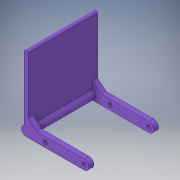
# Autodesk Inventor part: Mouth-Height-Lever-front
Saved by Autodesk Inventor 2018.3 (Build 223284000, 284)
## iProperties
Created: 2018-05-17
Part Number: Mouth-Height-Lever-front
Material: Generisch
Document SubType Name: Modeling
Designer: JochenAlt
Density: 1 g/cm^3
Appearance: Violett
Author: JochenAlt
Autodesk Inventor part; units mm, degrees
ref_plane "YZ Plane" through (0, 0, 0) normal (1, 0, 0) x (0, 1, 0)
ref_plane "XZ Plane" through (0, 0, 0) normal (0, 1, 0) x (-1, 0, 0)
ref_plane "XY Plane" through (0, 0, 0) normal (0, 0, 1) x (1, 0, 0)
sketch "Skizze4" plane through (0, 0, 0) normal (0, 1, 0) x (-1, 0, 0)
  line L0 (-32.5, 2.5) -> (-2.5, 2.5) construction
  line L1 (0, -10.2627) -> (0, 44.0763) construction
  line L2 (-42, 0) -> (7, 0) construction
  circle A0 centre (-32.5, 0) radius 2.5
  circle A1 centre (-32.5, 0) radius 1
  circle A2 centre (-2.5, 0) radius 2.5
  line L3 (-2.5, -2.5) -> (-32.5, -2.5) construction
  circle A3 centre (-12.5, 0) radius 2.5
  line L4 (-32.5, 2.5) -> (-12.5, 2.5)
  line L5 (-12.5, 2.5) -> (-7.7873, 2.5)
  line L6 (-32.5, -2.5) -> (-12.5, -2.5)
  line L7 (-12.5, -2.5) -> (-7.7873, -2.5)
  line L8 (-1.5, 2.2913) -> (-1.5, 35.3136)
  arc A4 (-1.5, 35.3136) -> (-3.5, 35.3136) centre (-2.5, 35.3136) ccw
  circle A5 centre (-12.5, 0) radius 1
  line L9 (-7.7873, 2.5) -> (-3.5, 6.3118)
  line L10 (-3.5, 6.3118) -> (-3.5, 35.3136)
  line L11 (-7.7873, 2.5) -> (-2.5, 2.5)
  line L12 (-7.7873, 2.5) -> (-7.7873, -2.5)
  line L13 (-7.7873, -2.5) -> (-2.5, -2.5)
  line L14 (-3.5, 6.3118) -> (-3.5, 2.2913)
  point P0 (0, 0)
  dimension "d28" = 2
  dimension "d30" = 10
  dimension "d32" = 20
  dimension "d33" = 5
  dimension "d35" = 5
  constraints: 26 end point, 16 point on circle, 9 tangent, 6 centre point, 5 parallel, 3 horizontal, 2 coincident, 2 vertical, 1 collinear, 1 equal radius, 2 other
  measures "d28" diameter of A1
  measures "d30" distance of A2.centre A3.centre
  measures "d32" distance of A3.centre A0.centre
  measures "d33" distance between parallel lines of L6 L4
  measures "d35" diameter of A2
extrude "Extrusion6" add sketch "Skizze4" along normal mid plane 36
extrude "Extrusion7" cut sketch "Skizze4" along normal mid plane 31 contours A0 | A0 L4 A3 L6 | L5 L12 L7 A3 | A3 | L9 L14 L11 | L11 L14 A2 L13 L12 | L11 A2 L14 | A1
sketch "Skizze2" plane through (2.5, -18.5, -2.6429) normal (0, -1, 0) x (1, 0, 0)
  circle A0 centre (51, 2.5) radius 1
  circle A1 centre (31, 2.5) radius 1
  arc A2 (-2.5, 2.5) -> (0, 0) centre (0, 2.5) ccw projected
  line L0 (-2.5, 5) -> (-2.5, 2.5) projected
  line L1 (-2.5, 5) -> (31.5, 5) construction
  arc A3 (51, 0) -> (51, 5) centre (51, 2.5) ccw projected
  point P0 (-2.5, 2.6429)
  point P1 (0, 5)
  dimension "d11" = 2
  dimension "d24" = 20
  constraints: 2 centre point, 1 concentric, 1 equal radius
  measures "d11" diameter of A0
  measures "d24" distance of A1.centre A0.centre
sketch "Skizze3" plane through (0, -15, 2.3571) normal (0, 0, 1) x (1, 0, 0)
  line L0 (0, -0.5) -> (0, -3.5) projected
  line L1 (53.5, 33.5) -> (0, 33.5) projected
  line L2 (0, -3.5) -> (2, -3.5)
  line L3 (2, -3.5) -> (2, 33.5)
  line L4 (2, 33.5) -> (0, 33.5)
  line L5 (0, 33.5) -> (0, -3.5)
  point P0 (0, 15)
  point P1 (29.5, 35.5)
  dimension "d14" = 2
  constraints: 8 end point, 2 parallel, 1 horizontal, 1 perpendicular, 2 other
  measures "d14" distance of L0.end L2.end
